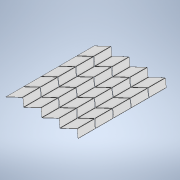
# Autodesk Inventor part: Part1
Saved by Autodesk Inventor 2020 (Build 240168000, 168)
## iProperties
Created: 2020-05-13
Part Number: Part1
Material: Generic
Document SubType Name: Modeling
Designer: maxde
Density: 1 g/cm^3
Appearance: Default
Author: maxde
Autodesk Inventor part; units mm, degrees
ref_plane "YZ Plane" through (0, 0, 0) normal (1, 0, 0) x (0, 1, 0)
ref_plane "XZ Plane" through (0, 0, 0) normal (0, 1, 0) x (-1, 0, 0)
ref_plane "XY Plane" through (0, 0, 0) normal (0, 0, 1) x (1, 0, 0)
sketch "Sketch1" plane through (0, 0, 0) normal (0, 1, 0) x (-1, 0, 0)
  line L0 (0, 0) -> (0, -47) construction
  line L1 (0, 0) -> (0, -22) construction
  line L2 (-24, -22) -> (0, 0) construction
  line L3 (-24, -22) -> (-24, -69) construction
  line L4 (-24, -69) -> (0, -47) construction
  line L5 (-0.675, -46.7031) -> (-0.675, -1.5344)
  line L6 (-0.675, -1.5344) -> (-23.325, -22.2969)
  line L7 (-23.325, -22.2969) -> (-23.325, -67.4656)
  line L8 (-23.325, -67.4656) -> (-0.675, -46.7031)
  line L9 (24, -22) -> (0, 0) construction
  line L10 (24, -22) -> (24, -69) construction
  line L11 (24, -69) -> (0, -47) construction
  line L12 (0.675, -46.7031) -> (0.675, -1.5344)
  line L13 (0.675, -1.5344) -> (23.325, -22.2969)
  line L14 (23.325, -22.2969) -> (23.325, -67.4656)
  line L15 (23.325, -67.4656) -> (0.675, -46.7031)
  line L16 (48, 0) -> (48, -47) construction
  line L17 (48, 0) -> (48, -22) construction
  line L18 (24, -22) -> (48, 0) construction
  line L19 (24, -22) -> (24, -69) construction
  line L20 (24, -69) -> (48, -47) construction
  line L21 (47.325, -46.7031) -> (47.325, -1.5344)
  line L22 (47.325, -1.5344) -> (24.675, -22.2969)
  line L23 (24.675, -22.2969) -> (24.675, -67.4656)
  line L24 (24.675, -67.4656) -> (47.325, -46.7031)
  line L25 (72, -22) -> (48, 0) construction
  line L26 (72, -22) -> (72, -69) construction
  line L27 (72, -69) -> (48, -47) construction
  line L28 (48.675, -46.7031) -> (48.675, -1.5344)
  line L29 (48.675, -1.5344) -> (71.325, -22.2969)
  line L30 (71.325, -22.2969) -> (71.325, -67.4656)
  line L31 (71.325, -67.4656) -> (48.675, -46.7031)
  line L32 (-48, 0) -> (-48, -47) construction
  line L33 (-72, -22) -> (-48, 0) construction
  line L34 (-72, -22) -> (-72, -69) construction
  line L35 (-72, -69) -> (-48, -47) construction
  line L36 (-48.675, -46.7031) -> (-48.675, -1.5344)
  line L37 (-48.675, -1.5344) -> (-71.325, -22.2969)
  line L38 (-71.325, -22.2969) -> (-71.325, -67.4656)
  line L39 (-71.325, -67.4656) -> (-48.675, -46.7031)
  line L40 (-24, -22) -> (-48, 0) construction
  line L41 (-24, -22) -> (-24, -69) construction
  line L42 (-24, -69) -> (-48, -47) construction
  line L43 (-47.325, -46.7031) -> (-47.325, -1.5344)
  line L44 (-47.325, -1.5344) -> (-24.675, -22.2969)
  line L45 (-24.675, -22.2969) -> (-24.675, -67.4656)
  line L46 (-24.675, -67.4656) -> (-47.325, -46.7031)
  line L47 (-24, -22) -> (-24, -69) construction
  line L48 (0, -47) -> (0, -94) construction
  line L49 (0, -47) -> (0, -69) construction
  line L50 (-24, -69) -> (0, -47) construction
  line L51 (-24, -69) -> (-24, -116) construction
  line L52 (-24, -116) -> (0, -94) construction
  line L53 (-0.675, -93.7031) -> (-0.675, -48.5344)
  line L54 (-0.675, -48.5344) -> (-23.325, -69.2969)
  line L55 (-23.325, -69.2969) -> (-23.325, -114.4656)
  line L56 (-23.325, -114.4656) -> (-0.675, -93.7031)
  line L57 (24, -69) -> (0, -47) construction
  line L58 (24, -69) -> (24, -116) construction
  line L59 (24, -116) -> (0, -94) construction
  line L60 (0.675, -93.7031) -> (0.675, -48.5344)
  line L61 (0.675, -48.5344) -> (23.325, -69.2969)
  line L62 (23.325, -69.2969) -> (23.325, -114.4656)
  line L63 (23.325, -114.4656) -> (0.675, -93.7031)
  line L64 (48, -47) -> (48, -69) construction
  line L65 (47.325, -48.5344) -> (24.675, -69.2969)
  line L66 (48.675, -93.7031) -> (48.675, -48.5344)
  line L67 (47.325, -93.7031) -> (47.325, -48.5344)
  line L68 (48, -47) -> (48, -94) construction
  line L69 (24, -69) -> (48, -47) construction
  line L70 (72, -69) -> (48, -47) construction
  line L71 (48.675, -48.5344) -> (71.325, -69.2969)
  line L72 (71.325, -114.4656) -> (48.675, -93.7031)
  line L73 (24.675, -114.4656) -> (47.325, -93.7031)
  line L74 (24.675, -69.2969) -> (24.675, -114.4656)
  line L75 (24, -69) -> (24, -116) construction
  line L76 (24, -116) -> (48, -94) construction
  line L77 (72, -116) -> (48, -94) construction
  line L78 (71.325, -69.2969) -> (71.325, -114.4656)
  line L79 (72, -69) -> (72, -116) construction
  line L80 (-24.675, -69.2969) -> (-24.675, -114.4656)
  line L81 (-24, -69) -> (-24, -116) construction
  line L82 (-24, -69) -> (-24, -116) construction
  line L83 (-24.675, -114.4656) -> (-47.325, -93.7031)
  line L84 (-24, -116) -> (-48, -94) construction
  line L85 (-71.325, -114.4656) -> (-48.675, -93.7031)
  line L86 (-72, -116) -> (-48, -94) construction
  line L87 (-71.325, -69.2969) -> (-71.325, -114.4656)
  line L88 (-72, -69) -> (-72, -116) construction
  line L89 (-48.675, -48.5344) -> (-71.325, -69.2969)
  line L90 (-72, -69) -> (-48, -47) construction
  line L91 (-47.325, -48.5344) -> (-24.675, -69.2969)
  line L92 (-24, -69) -> (-48, -47) construction
  line L93 (-48.675, -93.7031) -> (-48.675, -48.5344)
  line L94 (-47.325, -93.7031) -> (-47.325, -48.5344)
  line L95 (-48, -47) -> (-48, -94) construction
  line L96 (0, -94) -> (0, -141) construction
  line L97 (0, -94) -> (0, -116) construction
  line L98 (-24, -116) -> (0, -94) construction
  line L99 (-24, -116) -> (-24, -163) construction
  line L100 (-24, -163) -> (0, -141) construction
  line L101 (-0.675, -140.7031) -> (-0.675, -95.5344)
  line L102 (-0.675, -95.5344) -> (-23.325, -116.2969)
  line L103 (-23.325, -116.2969) -> (-23.325, -161.4656)
  line L104 (-23.325, -161.4656) -> (-0.675, -140.7031)
  line L105 (24, -116) -> (0, -94) construction
  line L106 (24, -116) -> (24, -163) construction
  line L107 (24, -163) -> (0, -141) construction
  line L108 (0.675, -140.7031) -> (0.675, -95.5344)
  line L109 (0.675, -95.5344) -> (23.325, -116.2969)
  line L110 (23.325, -116.2969) -> (23.325, -161.4656)
  line L111 (23.325, -161.4656) -> (0.675, -140.7031)
  line L112 (48, -94) -> (48, -116) construction
  line L113 (47.325, -95.5344) -> (24.675, -116.2969)
  line L114 (48.675, -140.7031) -> (48.675, -95.5344)
  line L115 (47.325, -140.7031) -> (47.325, -95.5344)
  line L116 (48, -94) -> (48, -141) construction
  line L117 (24, -116) -> (48, -94) construction
  line L118 (72, -116) -> (48, -94) construction
  line L119 (48.675, -95.5344) -> (71.325, -116.2969)
  line L120 (71.325, -161.4656) -> (48.675, -140.7031)
  line L121 (24.675, -161.4656) -> (47.325, -140.7031)
  line L122 (24.675, -116.2969) -> (24.675, -161.4656)
  line L123 (24, -116) -> (24, -163) construction
  line L124 (24, -163) -> (48, -141) construction
  line L125 (72, -163) -> (48, -141) construction
  line L126 (71.325, -116.2969) -> (71.325, -161.4656)
  line L127 (72, -116) -> (72, -163) construction
  line L128 (-24.675, -116.2969) -> (-24.675, -161.4656)
  line L129 (-24, -116) -> (-24, -163) construction
  line L130 (-24, -116) -> (-24, -163) construction
  line L131 (-24.675, -161.4656) -> (-47.325, -140.7031)
  line L132 (-24, -163) -> (-48, -141) construction
  line L133 (-71.325, -161.4656) -> (-48.675, -140.7031)
  line L134 (-72, -163) -> (-48, -141) construction
  line L135 (-71.325, -116.2969) -> (-71.325, -161.4656)
  line L136 (-72, -116) -> (-72, -163) construction
  line L137 (-48.675, -95.5344) -> (-71.325, -116.2969)
  line L138 (-72, -116) -> (-48, -94) construction
  line L139 (-47.325, -95.5344) -> (-24.675, -116.2969)
  line L140 (-24, -116) -> (-48, -94) construction
  line L141 (-48.675, -140.7031) -> (-48.675, -95.5344)
  line L142 (-47.325, -140.7031) -> (-47.325, -95.5344)
  line L143 (-48, -94) -> (-48, -141) construction
  line L144 (-71.325, -163.2969) -> (-71.325, -208.4656)
  line L145 (-71.325, -208.4656) -> (-48.675, -187.7031)
  line L146 (-72, -163) -> (-72, -210) construction
  line L147 (-72, -210) -> (-48, -188) construction
  line L148 (-24.675, -208.4656) -> (-47.325, -187.7031)
  line L149 (-24, -210) -> (-48, -188) construction
  line L150 (-24, -163) -> (-24, -210) construction
  line L151 (-24, -163) -> (-24, -210) construction
  line L152 (-24.675, -163.2969) -> (-24.675, -208.4656)
  line L153 (-47.325, -142.5344) -> (-24.675, -163.2969)
  line L154 (-24, -163) -> (-48, -141) construction
  line L155 (-47.325, -187.7031) -> (-47.325, -142.5344)
  line L156 (-48.675, -187.7031) -> (-48.675, -142.5344)
  line L157 (-48.675, -142.5344) -> (-71.325, -163.2969)
  line L158 (-72, -163) -> (-48, -141) construction
  line L159 (-48, -141) -> (-48, -188) construction
  line L160 (-0.675, -142.5344) -> (-23.325, -163.2969)
  line L161 (-24, -163) -> (0, -141) construction
  line L162 (0.675, -187.7031) -> (0.675, -142.5344)
  line L163 (0, -141) -> (0, -188) construction
  line L164 (0, -141) -> (0, -163) construction
  line L165 (0.675, -142.5344) -> (23.325, -163.2969)
  line L166 (24, -163) -> (0, -141) construction
  line L167 (-0.675, -187.7031) -> (-0.675, -142.5344)
  line L168 (24, -210) -> (0, -188) construction
  line L169 (23.325, -208.4656) -> (0.675, -187.7031)
  line L170 (24, -163) -> (24, -210) construction
  line L171 (24, -163) -> (24, -210) construction
  line L172 (23.325, -163.2969) -> (23.325, -208.4656)
  line L173 (24.675, -163.2969) -> (24.675, -208.4656)
  line L174 (24.675, -208.4656) -> (47.325, -187.7031)
  line L175 (24, -210) -> (48, -188) construction
  line L176 (71.325, -208.4656) -> (48.675, -187.7031)
  line L177 (72, -210) -> (48, -188) construction
  line L178 (71.325, -163.2969) -> (71.325, -208.4656)
  line L179 (72, -163) -> (72, -210) construction
  line L180 (-24, -163) -> (-24, -210) construction
  line L181 (-23.325, -208.4656) -> (-0.675, -187.7031)
  line L182 (-24, -210) -> (0, -188) construction
  line L183 (-23.325, -163.2969) -> (-23.325, -208.4656)
  line L184 (48.675, -142.5344) -> (71.325, -163.2969)
  line L185 (72, -163) -> (48, -141) construction
  line L186 (48.675, -187.7031) -> (48.675, -142.5344)
  line L187 (47.325, -187.7031) -> (47.325, -142.5344)
  line L188 (48, -141) -> (48, -188) construction
  line L189 (48, -141) -> (48, -163) construction
  line L190 (47.325, -142.5344) -> (24.675, -163.2969)
  line L191 (24, -163) -> (48, -141) construction
  line L192 (-72.675, -67.4656) -> (-95.325, -46.7031)
  line L193 (-72, -69) -> (-96, -47) construction
  line L194 (-72.675, -22.2969) -> (-72.675, -67.4656)
  line L195 (-95.325, -1.5344) -> (-72.675, -22.2969)
  line L196 (-72, -22) -> (-96, 0) construction
  line L197 (-95.325, -46.7031) -> (-95.325, -1.5344)
  line L198 (-96, 0) -> (-96, -47) construction
  line L199 (-72.675, -69.2969) -> (-72.675, -114.4656)
  line L200 (-72.675, -114.4656) -> (-95.325, -93.7031)
  line L201 (-72, -116) -> (-96, -94) construction
  line L202 (-95.325, -93.7031) -> (-95.325, -48.5344)
  line L203 (-95.325, -48.5344) -> (-72.675, -69.2969)
  line L204 (-72, -69) -> (-96, -47) construction
  line L205 (-96, -47) -> (-96, -94) construction
  line L206 (-72.675, -163.2969) -> (-72.675, -208.4656)
  line L207 (-72.675, -208.4656) -> (-95.325, -187.7031)
  line L208 (-72, -210) -> (-96, -188) construction
  line L209 (-95.325, -187.7031) -> (-95.325, -142.5344)
  line L210 (-96, -141) -> (-96, -188) construction
  line L211 (-96, -94) -> (-96, -141) construction
  line L212 (-95.325, -95.5344) -> (-72.675, -116.2969)
  line L213 (-72, -116) -> (-96, -94) construction
  line L214 (-95.325, -140.7031) -> (-95.325, -95.5344)
  line L215 (-95.325, -142.5344) -> (-72.675, -163.2969)
  line L216 (-72, -163) -> (-96, -141) construction
  line L217 (-72.675, -161.4656) -> (-95.325, -140.7031)
  line L218 (-72.675, -116.2969) -> (-72.675, -161.4656)
  line L219 (-72, -163) -> (-96, -141) construction
  line L220 (96, 0) -> (96, -22) construction
  line L221 (95.325, -46.7031) -> (95.325, -1.5344)
  line L222 (96, 0) -> (96, -47) construction
  line L223 (72, -22) -> (96, 0) construction
  line L224 (95.325, -1.5344) -> (72.675, -22.2969)
  line L225 (72.675, -67.4656) -> (95.325, -46.7031)
  line L226 (72, -69) -> (96, -47) construction
  line L227 (72.675, -22.2969) -> (72.675, -67.4656)
  line L228 (72.675, -114.4656) -> (95.325, -93.7031)
  line L229 (72, -116) -> (96, -94) construction
  line L230 (72.675, -69.2969) -> (72.675, -114.4656)
  line L231 (95.325, -48.5344) -> (72.675, -69.2969)
  line L232 (72, -69) -> (96, -47) construction
  line L233 (95.325, -93.7031) -> (95.325, -48.5344)
  line L234 (96, -47) -> (96, -94) construction
  line L235 (96, -47) -> (96, -69) construction
  line L236 (96, -141) -> (96, -188) construction
  line L237 (95.325, -187.7031) -> (95.325, -142.5344)
  line L238 (72.675, -208.4656) -> (95.325, -187.7031)
  line L239 (72, -210) -> (96, -188) construction
  line L240 (72.675, -163.2969) -> (72.675, -208.4656)
  line L241 (95.325, -95.5344) -> (72.675, -116.2969)
  line L242 (72, -116) -> (96, -94) construction
  line L243 (96, -94) -> (96, -116) construction
  line L244 (96, -94) -> (96, -141) construction
  line L245 (95.325, -140.7031) -> (95.325, -95.5344)
  line L246 (95.325, -142.5344) -> (72.675, -163.2969)
  line L247 (72, -163) -> (96, -141) construction
  line L248 (96, -141) -> (96, -163) construction
  line L249 (72.675, -161.4656) -> (95.325, -140.7031)
  line L250 (72.675, -116.2969) -> (72.675, -161.4656)
  line L251 (72, -163) -> (96, -141) construction
  line L252 (171.681, -198.7031) -> (171.681, -153.5344)
  line L253 (171.006, -152) -> (171.006, -199) construction
  line L254 (195.006, -174) -> (171.006, -152) construction
  line L255 (171.681, -153.5344) -> (194.331, -174.2969)
  line L256 (194.331, -219.4656) -> (171.681, -198.7031)
  line L257 (195.006, -221) -> (171.006, -199) construction
  line L258 (194.331, -174.2969) -> (194.331, -219.4656)
  line L259 (195.006, -174) -> (195.006, -221) construction
  line L260 (218.331, -198.7031) -> (218.331, -153.5344)
  line L261 (219.006, -152) -> (219.006, -199) construction
  line L262 (195.006, -174) -> (219.006, -152) construction
  line L263 (218.331, -153.5344) -> (195.681, -174.2969)
  line L264 (195.681, -219.4656) -> (218.331, -198.7031)
  line L265 (195.006, -221) -> (219.006, -199) construction
  line L266 (195.681, -174.2969) -> (195.681, -219.4656)
  line L267 (48, -188) -> (48, -235) construction
  line L268 (48.675, -234.7031) -> (48.675, -189.5344)
  line L269 (48.675, -189.5344) -> (71.325, -210.2969)
  line L270 (72, -210) -> (48, -188) construction
  line L271 (71.325, -255.4656) -> (48.675, -234.7031)
  line L272 (72, -257) -> (48, -235) construction
  line L273 (72, -210) -> (72, -257) construction
  line L274 (72.675, -210.2969) -> (72.675, -255.4656)
  line L275 (72.675, -255.4656) -> (95.325, -234.7031)
  line L276 (72, -257) -> (96, -235) construction
  line L277 (72, -210) -> (96, -188) construction
  line L278 (95.325, -189.5344) -> (72.675, -210.2969)
  line L279 (95.325, -234.7031) -> (95.325, -189.5344)
  line L280 (96, -188) -> (96, -235) construction
  line L281 (71.325, -210.2969) -> (71.325, -255.4656)
  line L282 (0, -188) -> (0, -235) construction
  line L283 (0.675, -234.7031) -> (0.675, -189.5344)
  line L284 (0.675, -189.5344) -> (23.325, -210.2969)
  line L285 (24, -210) -> (0, -188) construction
  line L286 (23.325, -255.4656) -> (0.675, -234.7031)
  line L287 (24, -257) -> (0, -235) construction
  line L288 (24, -210) -> (24, -257) construction
  line L289 (24.675, -210.2969) -> (24.675, -255.4656)
  line L290 (24.675, -255.4656) -> (47.325, -234.7031)
  line L291 (24, -257) -> (48, -235) construction
  line L292 (24, -210) -> (48, -188) construction
  line L293 (47.325, -189.5344) -> (24.675, -210.2969)
  line L294 (47.325, -234.7031) -> (47.325, -189.5344)
  line L295 (48, -188) -> (48, -235) construction
  line L296 (23.325, -210.2969) -> (23.325, -255.4656)
  line L297 (-48, -188) -> (-48, -235) construction
  line L298 (-47.325, -234.7031) -> (-47.325, -189.5344)
  line L299 (-47.325, -189.5344) -> (-24.675, -210.2969)
  line L300 (-24, -210) -> (-48, -188) construction
  line L301 (-24.675, -255.4656) -> (-47.325, -234.7031)
  line L302 (-24, -257) -> (-48, -235) construction
  line L303 (-24, -210) -> (-24, -257) construction
  line L304 (-23.325, -210.2969) -> (-23.325, -255.4656)
  line L305 (-23.325, -255.4656) -> (-0.675, -234.7031)
  line L306 (-24, -257) -> (0, -235) construction
  line L307 (-24, -210) -> (0, -188) construction
  line L308 (-0.675, -189.5344) -> (-23.325, -210.2969)
  line L309 (-0.675, -234.7031) -> (-0.675, -189.5344)
  line L310 (0, -188) -> (0, -235) construction
  line L311 (-24.675, -210.2969) -> (-24.675, -255.4656)
  line L312 (-96, -188) -> (-96, -235) construction
  line L313 (-95.325, -234.7031) -> (-95.325, -189.5344)
  line L314 (-95.325, -189.5344) -> (-72.675, -210.2969)
  line L315 (-72, -210) -> (-96, -188) construction
  line L316 (-72.675, -255.4656) -> (-95.325, -234.7031)
  line L317 (-72, -257) -> (-96, -235) construction
  line L318 (-72, -210) -> (-72, -257) construction
  line L319 (-71.325, -210.2969) -> (-71.325, -255.4656)
  line L320 (-71.325, -255.4656) -> (-48.675, -234.7031)
  line L321 (-72, -257) -> (-48, -235) construction
  line L322 (-72, -210) -> (-48, -188) construction
  line L323 (-48.675, -189.5344) -> (-71.325, -210.2969)
  line L324 (-48.675, -234.7031) -> (-48.675, -189.5344)
  line L325 (-48, -188) -> (-48, -235) construction
  line L326 (-72.675, -210.2969) -> (-72.675, -255.4656)
  point P0 (-48, -22)
  point P1 (-48, -69)
  point P2 (-48, -116)
  point P3 (-48, -163)
  point P4 (-96, -22)
  point P5 (-96, -69)
  point P6 (-96, -163)
  point P7 (-96, -116)
  dimension "d0" = 47
  dimension "d1" = 22
  dimension "d2" = 24
  dimension "d3" = 47
  dimension "d4" = 0.675
  dimension "d5" = 47
  dimension "d6" = 22
  dimension "d7" = 24
  dimension "d8" = 47
  dimension "d9" = 0.675
  dimension "d10" = 47
  dimension "d11" = 22
  dimension "d12" = 24
  dimension "d13" = 47
  dimension "d14" = 0.675
  dimension "d15" = 47
  dimension "d16" = 47
  dimension "d17" = 22
  dimension "d18" = 24
  dimension "d19" = 47
  dimension "d20" = 0.675
  dimension "d21" = 47
  dimension "d22" = 22
  dimension "d23" = 24
  dimension "d24" = 47
  dimension "d25" = 0.675
  dimension "d26" = 47
  dimension "d27" = 22
  dimension "d28" = 24
  dimension "d29" = 47
  dimension "d30" = 0.675
  dimension "d31" = 47
  dimension "d32" = 47
  dimension "d33" = 22
  dimension "d34" = 24
  dimension "d35" = 47
  dimension "d36" = 0.675
  dimension "d37" = 47
  dimension "d38" = 22
  dimension "d39" = 24
  dimension "d40" = 47
  dimension "d41" = 0.675
  dimension "d42" = 47
  dimension "d43" = 22
  dimension "d44" = 24
  dimension "d45" = 47
  dimension "d46" = 0.675
  dimension "d47" = 47
  dimension "d48" = 47
  dimension "d49" = 22
  dimension "d50" = 24
  dimension "d51" = 47
  dimension "d52" = 0.675
  dimension "d53" = 47
  dimension "d54" = 22
  dimension "d55" = 24
  dimension "d56" = 47
  dimension "d57" = 0.675
  dimension "d58" = 47
  dimension "d59" = 22
  dimension "d60" = 24
  dimension "d61" = 47
  dimension "d62" = 0.675
  dimension "d63" = 47
  constraints: 654 end point, 128 symmetric about line, 20 point on line, 17 vertical, 36 other
  measures "d0" distance of L0.start L0.end
  measures "d1" distance of L0.start L1.end
  measures "d2" distance of L1.end L2.start
  measures "d3" distance of L2.start L3.end
  measures "d4" distance between parallel lines of L0 L5
  measures "d5" distance of L17.start L16.end
  measures "d6" distance of L17.start L17.end
  measures "d7" distance of L17.end L18.start
  measures "d8" distance of L18.start L19.end
  measures "d9" distance between parallel lines of L16 L21
  measures "d10" distance of L33.end L42.end
  measures "d11" distance of L33.end point (-48, -22)
  measures "d12" distance of point (-48, -22) L34.start
  measures "d13" distance of L34.start L35.start
  measures "d14" distance between parallel lines of L32 L36
  measures "d15" distance of L47.start L47.end
  measures "d16" distance of L50.end L48.end
  measures "d17" distance of L50.end L49.end
  measures "d18" distance of L49.end L50.start
  measures "d19" distance of L50.start L51.end
  measures "d20" distance between parallel lines of L48 L53
  measures "d21" distance of L70.end L76.end
  measures "d22" distance of L70.end L64.end
  measures "d23" distance of L64.end L75.start
  measures "d24" distance of L75.start L75.end
  measures "d25" distance between parallel lines of L68 L67
  measures "d26" distance of L92.end L86.end
  measures "d27" distance of L92.end point (-48, -69)
  measures "d28" distance of point (-48, -69) L88.start
  measures "d29" distance of L88.start L88.end
  measures "d30" distance between parallel lines of L95 L93
  measures "d31" distance of L81.start L81.end
  measures "d32" distance of L105.end L100.end
  measures "d33" distance of L105.end L97.end
  measures "d34" distance of L97.end L99.start
  measures "d35" distance of L99.start L100.start
  measures "d36" distance between parallel lines of L96 L101
  measures "d37" distance of L118.end L116.end
  measures "d38" distance of L118.end L112.end
  measures "d39" distance of L112.end L123.start
  measures "d40" distance of L123.start L123.end
  measures "d41" distance between parallel lines of L116 L115
  measures "d42" distance of L143.start L143.end
  measures "d43" distance of L143.start point (-48, -116)
  measures "d44" distance of point (-48, -116) L138.start
  measures "d45" distance of L138.start L134.start
  measures "d46" distance between parallel lines of L143 L141
  measures "d47" distance of L129.start L129.end
  measures "d48" distance of L163.start L163.end
  measures "d49" distance of L163.start L164.end
  measures "d50" distance of L164.end L180.start
  measures "d51" distance of L180.start L180.end
  measures "d52" distance between parallel lines of L163 L167
  measures "d53" distance of L188.start L188.end
  measures "d54" distance of L188.start L189.end
  measures "d55" distance of L189.end L171.start
  measures "d56" distance of L171.start L171.end
  measures "d57" distance between parallel lines of L188 L187
  measures "d58" distance of L159.start L149.end
  measures "d59" distance of L159.start point (-48, -163)
  measures "d60" distance of point (-48, -163) L146.start
  measures "d61" distance of L146.start L146.end
  measures "d62" distance between parallel lines of L159 L156
  measures "d63" distance of L150.start L150.end
extrude "Extrusion1" add sketch "Sketch1" along normal blind 0.6 contours L8 L7 L6 L5 | L12 L13 L14 L15 | L24 L23 L22 L21 | L28 L29 L30 L31 | L39 L38 L37 L36 | L43 L44 L45 L46 | L56 L55 L54 L53 | L60 L61 L62 L63 | L67 L73 L74 L65 | L66 L71 L78 L72 | L80 L83 L94 L91 | L87 L89 L93 L85 | L104 L103 L102 L101 | L108 L109 L110 L111 | L115 L121 L122 L113 | L114 L119 L126 L120 | L128 L131 L142 L139 | L135 L137 L141 L133 | L157 L156 L145 L144 | L148 L155 L153 L152 | L167 L181 L183 L160 | L162 L165 L172 L169 | L190 L187 L174 L173 | L176 L186 L184 L178 | L192 L197 L195 L194 | L199 L200 L202 L203 | L206 L207 L209 L215 | L212 L218 L217 L214 | L225 L227 L224 L221 | L230 L231 L233 L228 | L238 L240 L246 L237 | L245 L249 L250 L241 | L268 L269 L281 L271 | L278 L279 L275 L274 | L283 L284 L296 L286 | L293 L294 L290 L289 | L298 L299 L311 L301 | L308 L309 L305 L304 | L313 L314 L326 L316 | L323 L324 L320 L319
body "Solid1"
